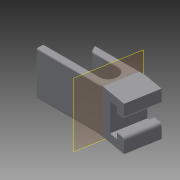
# Autodesk Inventor part: pinza0.3
Saved by Autodesk Inventor 2015 SP1 (Build 190203100, 203)
## iProperties
Created: 2015-12-16
Part Number: pinza0.3
Material: Generic
Document SubType Name: Modeling
Designer: pc
Density: 1 g/cm^3
Appearance: Default
Author: pc
Autodesk Inventor part; units mm, degrees
ref_plane "YZ Plane" through (0, 0, 0) normal (1, 0, 0) x (0, 1, 0)
ref_plane "XZ Plane" through (0, 0, 0) normal (0, 1, 0) x (-1, 0, 0)
ref_plane "XY Plane" through (0, 0, 0) normal (0, 0, 1) x (1, 0, 0)
sketch "Sketch1" plane through (0, 0, 0) normal (0, 0, 1) x (1, 0, 0)
  line L0 (-25, 2.5) -> (-2.5, 2.5)
  line L1 (-2.5, 2.5) -> (-2.5, 8.5)
  line L2 (-2.5, 8.5) -> (-14.2044, 8.5)
  line L3 (-15.6271, 11) -> (0, 11)
  line L4 (0, 11) -> (0, 0)
  line L5 (0, 0) -> (-25, 0)
  line L6 (-25, 2.5) -> (-25, 0)
  line L7 (-15.6271, 11) -> (-14.2044, 8.5)
  dimension "d4" = 6
  dimension "d5" = 25
  dimension "d22" = 15.6271
  dimension "d23" = 11
  dimension "d24" = 11.7044
  dimension "d25" = 2.5
  constraints: 16 end point, 2 perpendicular, 1 coincident, 1 horizontal, 1 vertical, 2 other
  measures "d4" distance of L0.end L1.end
  measures "d5" distance of L4.end L5.end
  measures "d22" distance of L3.start L3.end
  measures "d23" distance of L3.end L4.end
  measures "d24" distance of L1.end L2.end
  measures "d25" distance of L0.start L5.end
extrude "Extrusion1" add sketch "Sketch1" along normal blind 15
ref_plane "Work Plane1" through (0, 11, 0) normal (0.9848078, -0.1736482, 0) x (0, 0, 1)
sketch "Sketch3" plane through (0, 0, 0) normal (0, 0, -1) x (-1, 0, 0)
  line L0 (3.1619, -6.9323) -> (-0.527, 13.9887) projected
  line L1 (25, 2.5) -> (2.5, 2.5) projected
  line L2 (2.5, 2.5) -> (2.5, 8.5) projected
  line L3 (2.5, 8.5) -> (14.2044, 8.5) projected
  line L4 (15.6271, 11) -> (0, 11) projected
  line L5 (0, 11) -> (0, 0) projected
  line L6 (0, 0) -> (25, 0) projected
  line L7 (25, 0) -> (25, 2.5) projected
  line L8 (25, 0) -> (0, 0) projected
  line L9 (1.9396, 0) -> (0, 0)
  line L10 (0, 0) -> (0, 11)
  line L11 (0, 11) -> (1.9396, 0)
  line L12 (14.2044, 8.5) -> (15.6271, 11) projected
  constraints: 6 end point, 2 point on line, 1 collinear, 1 perpendicular
extrude "Extrusion2" cut sketch "Sketch3" against normal blind 20 contours L6 L5 L0
sketch "Sketch4" plane through (-1.4988, 2.5, 15) normal (0.9848078, -0.1736482, 0) x (0, 0, 1)
  line L0 (0, 2.5386) -> (0, -8.6311) projected
  line L1 (-15, 2.5386) -> (0, 2.5386) projected
  line L2 (-15, -8.6311) -> (-15, 2.5386) projected
  line L3 (-15, -8.6311) -> (-15, 2.5386) projected
  line L4 (-15, -8.6311) -> (0, -8.6311) projected
  line L5 (0, 2.5386) -> (0, -8.6311) projected
  line L6 (-15, 2.5386) -> (-15, -8.6311)
  line L7 (-15, -8.6311) -> (0, -8.6311)
  line L8 (0, -8.6311) -> (0, 2.5386)
  line L9 (-15, 2.5386) -> (0, 2.5386) projected
  line L10 (-15, -8.6311) -> (0, -8.6311) projected
  point P0 (-15, 2.2018)
  constraints: 6 end point, 1 collinear, 1 perpendicular, 1 vertical
extrude "Extrusion3" add sketch "Sketch4" along normal blind 1
sketch "Sketch6" plane through (-1.9396, 0, 0) normal (-0.1736482, -0.9848078, 0) x (0.9848078, -0.1736482, 0)
  line L0 (1, 15) -> (1, 0) projected
  line L1 (1, 15) -> (9, 15)
  line L2 (9, 15) -> (9, 10.3)
  line L3 (9, 10.3) -> (6, 10.3)
  line L4 (6, 10.3) -> (6, 12.3)
  line L5 (6, 12.3) -> (3, 12.3)
  line L6 (3, 12.3) -> (3, 2.7)
  line L7 (3, 2.7) -> (6, 2.7)
  line L8 (6, 2.7) -> (6, 4.7)
  line L9 (6, 4.7) -> (9, 4.7)
  line L10 (9, 4.7) -> (9, 0)
  line L11 (9, 0) -> (1, 0)
  line L12 (1, 0) -> (1, 15)
  point P0 (1.9101, 0)
  dimension "d13" = 5.6
  dimension "d14" = 2
  dimension "d15" = 2
  dimension "d16" = 3
  dimension "d17" = 3
  constraints: 24 end point, 9 perpendicular, 4 point on line, 2 collinear, 1 horizontal
  measures "d13" distance of L9.end L2.end
  measures "d14" distance of L3.end L4.end
  measures "d15" distance between parallel lines of L0 L6
  measures "d16" distance of L6.end L7.end
  measures "d17" distance of L8.end L9.end
extrude "Extrusion4" add sketch "Sketch6" against normal up to surface (11.1697 mm away)
fillet "Fillet3" radius 1 2 edges at (7.8935, 3.9372, 4.7) (7.8935, 3.9372, 10.3)
fillet "Fillet1" radius 2.8 2 edges at (-2.5, 2.5, 7.5) (-2.5, 8.5, 7.5)
fillet "Fillet2" radius 0.5 20 edges at (-15.15, 2.5, 0) (-25, 2.5, 7.5) (-15.15, 2.5, 15) (-9.7522, 8.5, 15) (-14.2044, 8.5, 7.5) (-9.7522, 8.5, 0) (-15.6271, 11, 7.5) (-7.8135, 11, 0) (-7.8135, 11, 15) (-13.4698, 0, 0) (-13.4698, 0, 15) (-25, 0, 7.5) (-25, 1.25, 0) (-25, 1.25, 15) (-3.3201, 3.3201, 0) (-3.3201, 3.3201, 15) (-2.5, 5.5, 0) (-2.5, 5.5, 15) (-3.3201, 7.6799, 0) (-3.3201, 7.6799, 15)
body "Solid1"
